Blumal_keks v1_v2 (Autodesk Fusion 360 design; units mm, degrees)
Autodesk Fusion 360 part; units mm, degrees
sketch "Skizze2" plane through (0, 0, 0) normal (0, 1, 0) x (1, 0, 0)
  arc A0 (62.9864, 7.1267) -> (58.1355, 7.7875) centre (59.7342, 1.3882) ccw
  arc A1 (70.9784, 31.7234) -> (68.8509, 27.3141) centre (75.431, 26.8571) ccw
  arc A2 (31.2594, 27.3141) -> (29.1319, 31.7234) centre (24.6793, 26.8571) ccw
  arc A3 (66.6655, 34.0402) -> (70.9784, 31.7234) centre (71.7203, 38.2775) ccw
  arc A4 (38.3975, 21.1373) -> (36.616, 11.2834) centre (43.0017, 15.2169) ccw
  arc A5 (63.857, 11.9444) -> (62.9864, 7.1267) centre (69.449, 8.4464) ccw
  arc A6 (50.0552, 46.9251) -> (53.5913, 43.5391) centre (56.0592, 49.656) ccw
  arc A7 (31.1643, 28.0621) -> (38.3975, 21.1373) centre (38.6425, 28.6333) ccw
  arc A8 (63.4943, 11.2834) -> (61.7128, 21.1373) centre (57.1086, 15.2169) ccw
  arc A9 (47.201, 43.8608) -> (42.8503, 34.8416) centre (50.0552, 36.9251) ccw
  arc A10 (57.26, 34.8416) -> (52.9093, 43.8608) centre (50.0552, 36.9251) ccw
  arc A11 (46.519, 43.5391) -> (50.0552, 46.9251) centre (44.0511, 49.656) ccw
  arc A12 (61.7128, 21.1373) -> (68.9461, 28.0621) centre (61.4678, 28.6333) ccw
  arc A13 (41.2341, 7.9281) -> (50.0552, 12.6675) centre (43.0017, 15.2169) ccw
  arc A14 (42.8503, 34.8416) -> (32.9282, 33.4909) centre (38.6425, 28.6333) ccw
  arc A15 (67.1821, 33.4909) -> (57.26, 34.8416) centre (61.4678, 28.6333) ccw
  arc A16 (37.1239, 7.1267) -> (36.2533, 11.9444) centre (30.6613, 8.4464) ccw
  arc A17 (29.1319, 31.7234) -> (33.4448, 34.0402) centre (28.39, 38.2775) ccw
  arc A18 (41.9748, 7.7875) -> (37.1239, 7.1267) centre (40.3761, 1.3882) ccw
  arc A19 (50.0552, 12.6675) -> (58.8762, 7.9281) centre (57.1086, 15.2169) ccw
  arc A20 (29.5468, 31.588) -> (33.7739, 33.8587) centre (28.8197, 38.0117) ccw
  arc A21 (62.7276, 7.4808) -> (57.9732, 8.1284) centre (59.5401, 1.8565) ccw
  arc A22 (41.4081, 8.2663) -> (50.0537, 12.9113) centre (43.1406, 15.4099) ccw
  arc A23 (50.0537, 12.9113) -> (58.6992, 8.2663) centre (56.9667, 15.4099) ccw
  arc A24 (42.1342, 8.1284) -> (37.3797, 7.4808) centre (40.5672, 1.8565) ccw
  arc A25 (47.2563, 43.4838) -> (42.9922, 34.6442) centre (50.0537, 36.6861) ccw
  arc A26 (63.5809, 12.2026) -> (62.7276, 7.4808) centre (69.0616, 8.7742) ccw
  arc A27 (31.5387, 27.9995) -> (38.628, 21.2125) centre (38.8681, 28.5594) ccw
  arc A28 (66.3334, 33.8587) -> (70.5605, 31.588) centre (71.2877, 38.0117) ccw
  arc A29 (42.9922, 34.6442) -> (33.2675, 33.3204) centre (38.8681, 28.5594) ccw
  arc A30 (70.5605, 31.588) -> (68.4754, 27.2664) centre (74.9245, 26.8186) ccw
  arc A31 (61.4793, 21.2125) -> (68.5686, 27.9995) centre (61.2392, 28.5594) ccw
  arc A32 (31.6319, 27.2664) -> (29.5468, 31.588) centre (25.1828, 26.8186) ccw
  arc A33 (38.628, 21.2125) -> (36.8819, 11.5547) centre (43.1406, 15.4099) ccw
  arc A34 (46.5879, 43.1686) -> (50.0537, 46.4871) centre (44.1691, 49.1637) ccw
  arc A35 (57.1151, 34.6442) -> (52.851, 43.4838) centre (50.0537, 36.6861) ccw
  arc A36 (50.0537, 46.4871) -> (53.5194, 43.1686) centre (55.9382, 49.1637) ccw
  arc A37 (66.8398, 33.3204) -> (57.1151, 34.6442) centre (61.2392, 28.5594) ccw
  arc A38 (37.3797, 7.4808) -> (36.5265, 12.2026) centre (31.0458, 8.7742) ccw
  arc A39 (63.2254, 11.5547) -> (61.4793, 21.2125) centre (56.9667, 15.4099) ccw
extrude "Extrusion1" add sketch "Skizze2" along normal blind 17 contours A0 A1 A2 A3 A4 A5 A6 A7 A8 A9 A10 A11 A12 A13 A14 A15 A16 A17 A18 A19 makes body 1
mirror "Spiegeln1" about plane through (0, 0, 0) normal (1, 0, 0) of bodies 1 makes body 2
move_body "Körper bewegen1" bodies 2 to x (1, 0, 0) y (0, 1, 0) z (0, 0, 1) at (59, 0, 0)
copy_body "Körper kopieren/einfügen1" bodies 1 makes body 3
move_body "Körper bewegen2" bodies 3 to x (1, 0, 0) y (0, 1, 0) z (0, 0, 1) at (-82, 0, 0)
copy_body "Körper kopieren/einfügen2" bodies 1 2 3 makes body 4 makes body 5 makes body 6
move_body "Körper bewegen3" bodies 4 5 6 to x (1, 0, 0) y (0, 1, 0) z (0, 0, 1) at (0, 0, -34.5)
sketch "Skizze3" plane through (0, 0, 0) normal (0, 1, 0) x (1, 0, 0)
  line L0 (70, 5) -> (65, 5)
  line L1 (65, 5) -> (65, 81)
  line L2 (65, 81) -> (70, 81)
  line L3 (70, 81) -> (70, 5)
  line L4 (70, 81) -> (-53, 81)
  line L5 (-53, 81) -> (-53, 76)
  line L6 (-53, 76) -> (70, 76)
  line L7 (70, 76) -> (70, 81)
  dimension "d4" = 76
  dimension "d5" = 5
  dimension "d6" = 123
  dimension "d7" = 5
  constraint horizontal L0
  constraint vertical L1
  constraint horizontal L2
  constraint vertical L3
  constraint horizontal L4
  constraint vertical L5
  constraint horizontal L6
  constraint vertical L7
  measures "d4" distance of L0.start L2.end
  measures "d5" distance of L0.start L0.end
  measures "d6" distance of L2.end L4.end
  measures "d7" distance of L2.end L6.end
extrude "Extrusion2" cut sketch "Skizze3" along normal blind 3 bodies 1 4 5 6
extrude "Extrusion3" add sketch "Skizze3" along normal blind 3 separate body makes body 7
copy_body "Körper kopieren/einfügen4" bodies 7 makes body 8
move_body "Körper bewegen5" bodies 8 to x (-1, 0, 0) y (0, 1, 0) z (0, 0, -1) at (17, 0, -86)
copy_body "Körper->Berechn1" bodies 1 removing the originals makes body 9 in component "Component"
copy_body "Körper->Berechn2" bodies 2 removing the originals makes body 10 in component "Component'"
copy_body "Körper->Berechn3" bodies 7 removing the originals makes body 11 in component "Component''"
copy_body "Körper->Berechn4" bodies 3 removing the originals makes body 12 in component "Component'''"
copy_body "Körper->Berechn5" bodies 4 removing the originals makes body 13 in component "Component''''"
copy_body "Körper->Berechn6" bodies 5 removing the originals makes body 14 in component "Component'''''"
copy_body "Körper->Berechn7" bodies 6 removing the originals makes body 15 in component "Component''''''"
copy_body "Körper->Berechn8" bodies 8 removing the originals makes body 16 in component "Component'''''''"
component "Component" placed x (1, 0, 0) y (0, 1, 0) z (0, 0, 1) at (0, 0, 0)
component "Component'" placed x (1, 0, 0) y (0, 1, 0) z (0, 0, 1) at (0, 0, 0)
component "Component''" placed x (1, 0, 0) y (0, 1, 0) z (0, 0, 1) at (0, 0, 0)
component "Component'''" placed x (1, 0, 0) y (0, 1, 0) z (0, 0, 1) at (0, 0, 0)
component "Component''''" placed x (1, 0, 0) y (0, 1, 0) z (0, 0, 1) at (0, 0, 0)
component "Component'''''" placed x (1, 0, 0) y (0, 1, 0) z (0, 0, 1) at (0, 0, 0)
component "Component''''''" placed x (1, 0, 0) y (0, 1, 0) z (0, 0, 1) at (0, 0, 0)
component "Component'''''''" placed x (1, 0, 0) y (0, 1, 0) z (0, 0, 1) at (0, 0, 0)
